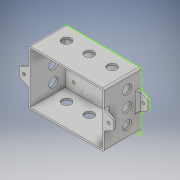
# Autodesk Inventor part: Contenedor Puente H v1.1
Saved by Autodesk Inventor 2019 (Build 230136000, 136)
## iProperties
Created: 2018-07-23
Part Number: Contenedor Puente H v1.1
Material: Genérico
Document SubType Name: Modeling
Designer: Francisco
Density: 1 g/cm^3
Appearance: Valor por defecto
Author: Francisco
Autodesk Inventor part; units mm, degrees
ref_plane "YZ Plane" through (0, 0, 0) normal (1, 0, 0) x (0, 1, 0)
ref_plane "XZ Plane" through (0, 0, 0) normal (0, 1, 0) x (-1, 0, 0)
ref_plane "XY Plane" through (0, 0, 0) normal (0, 0, 1) x (1, 0, 0)
sketch "Base" plane through (0, 0, 0) normal (0, 0, 1) x (1, 0, 0)
  line L0 (-41.5, -30) -> (41.5, -30)
  line L1 (41.5, -30) -> (41.5, -11.2361)
  line L2 (41.5, 30) -> (-41.5, 30)
  line L3 (-41.5, -30) -> (41.5, 30) construction
  line L4 (41.5, -30) -> (-41.5, 30) construction
  line L5 (-39.5, -28) -> (39.5, -28)
  line L6 (39.5, -28) -> (39.5, 28)
  line L7 (39.5, 28) -> (-39.5, 28)
  line L8 (-39.5, 28) -> (-39.5, -28)
  circle A0 centre (-30, -18.5) radius 1.35
  circle A1 centre (30, -18.5) radius 1.35
  circle A2 centre (0, 18.5) radius 1.35
  line L9 (51.5, 3.7639) -> (51.5, -3.7639)
  line L10 (41.5, 5) -> (51.5, -5) construction
  line L11 (51.5, 5) -> (41.5, -5) construction
  line L12 (42.6056, -9.4472) -> (50.3944, -5.5528)
  line L13 (50.3944, 5.5528) -> (42.6056, 9.4472)
  arc A3 (51.5, 3.7639) -> (50.3944, 5.5528) centre (49.5, 3.7639) ccw
  arc A4 (50.3944, -5.5528) -> (51.5, -3.7639) centre (49.5, -3.7639) ccw
  arc A5 (42.6056, -9.4472) -> (41.5, -11.2361) centre (43.5, -11.2361) ccw
  line L14 (41.5, 11.2361) -> (41.5, 30)
  arc A6 (41.5, 11.2361) -> (42.6056, 9.4472) centre (43.5, 11.2361) ccw
  line L15 (-41.5, -30) -> (-41.5, -11.2361)
  line L16 (-39.5, -28) -> (-39.5, 28)
  line L17 (-51.5, 3.7639) -> (-51.5, -3.7639)
  line L18 (-41.5, 5) -> (-51.5, -5) construction
  line L19 (-51.5, 5) -> (-41.5, -5) construction
  line L20 (-42.6056, -9.4472) -> (-50.3944, -5.5528)
  line L21 (-50.3944, 5.5528) -> (-42.6056, 9.4472)
  arc A7 (-50.3944, 5.5528) -> (-51.5, 3.7639) centre (-49.5, 3.7639) ccw
  arc A8 (-51.5, -3.7639) -> (-50.3944, -5.5528) centre (-49.5, -3.7639) ccw
  arc A9 (-41.5, -11.2361) -> (-42.6056, -9.4472) centre (-43.5, -11.2361) ccw
  line L22 (-41.5, 11.2361) -> (-41.5, 30)
  arc A10 (-42.6056, 9.4472) -> (-41.5, 11.2361) centre (-43.5, 11.2361) ccw
  line L23 (41.5, 11.2361) -> (41.5, -11.2361)
  line L24 (-41.5, -11.2361) -> (-41.5, 11.2361)
  circle A11 centre (-46.5, 0) radius 1.35
  circle A12 centre (46.5, 0) radius 1.35
  line L25 (-41.5, -34) -> (41.5, -34)
  line L26 (41.5, -34) -> (41.5, -11.2361)
  line L27 (41.5, 30) -> (-41.5, 30)
  line L28 (-41.5, -34) -> (41.5, 30) construction
  line L29 (41.5, -34) -> (-41.5, 30) construction
  line L30 (-39.5, -28) -> (35.5, -28)
  line L31 (35.5, -28) -> (35.5, 24)
  line L32 (35.5, 24) -> (-39.5, 24)
  line L33 (-39.5, 24) -> (-39.5, -28)
  circle A13 centre (-30, -18.5) radius 1.35
  circle A14 centre (30, -18.5) radius 1.35
  line L34 (51.5, 3.7639) -> (51.5, -3.7639)
  line L35 (41.5, 5) -> (51.5, -5) construction
  line L36 (51.5, 5) -> (41.5, -5) construction
  line L37 (42.6056, -9.4472) -> (50.3944, -5.5528)
  line L38 (50.3944, 5.5528) -> (42.6056, 9.4472)
  arc A15 (51.5, 3.7639) -> (50.3944, 5.5528) centre (49.5, 3.7639) ccw
  arc A16 (50.3944, -5.5528) -> (51.5, -3.7639) centre (49.5, -3.7639) ccw
  arc A17 (42.6056, -9.4472) -> (41.5, -11.2361) centre (43.5, -11.2361) ccw
  line L39 (41.5, 11.2361) -> (41.5, 30)
  arc A18 (41.5, 11.2361) -> (42.6056, 9.4472) centre (43.5, 11.2361) ccw
  line L40 (-51.5, -0.2361) -> (-51.5, -7.7639)
  line L41 (-41.5, 1) -> (-51.5, -9) construction
  line L42 (-51.5, 1) -> (-41.5, -9) construction
  arc A19 (-50.3944, 1.5528) -> (-51.5, -0.2361) centre (-49.5, -0.2361) ccw
  line L43 (-50.3944, 1.5528) -> (-42.6056, 5.4472)
  arc A20 (-42.6056, 5.4472) -> (-41.5, 7.2361) centre (-43.5, 7.2361) ccw
  line L44 (-41.5, 7.2361) -> (-41.5, 30)
  arc A21 (-51.5, -7.7639) -> (-50.3944, -9.5528) centre (-49.5, -7.7639) ccw
  line L45 (-42.6056, -13.4472) -> (-50.3944, -9.5528)
  arc A22 (-41.5, -15.2361) -> (-42.6056, -13.4472) centre (-43.5, -15.2361) ccw
  line L46 (-41.5, -34) -> (-41.5, -15.2361)
  line L47 (-39.5, -28) -> (-39.5, 24)
  line L48 (41.5, 11.2361) -> (41.5, -11.2361)
  line L49 (-41.5, -15.2361) -> (-41.5, 7.2361)
  circle A23 centre (-46.5, -4) radius 1.35
  circle A24 centre (46.5, 0) radius 1.35
  circle A25 centre (0, 18.5) radius 1.6
  circle A26 centre (30, -18.5) radius 1.6
  circle A27 centre (-30, -18.5) radius 1.6
  circle A28 centre (-46.5, 0) radius 1.6
  circle A29 centre (46.5, 0) radius 1.6
  point P0 (0, 0)
  point P1 (41.5, 10)
  point P2 (-41.5, 10)
  point P3 (-41.5, -10)
  point P4 (-41.5, 10)
  point P5 (0, -2)
  point P6 (41.5, 10)
  point P7 (-41.5, 10)
  point P8 (-41.5, -10)
  point P9 (-41.5, 6)
  dimension "d0" = 83
  dimension "d1" = 60
  dimension "d5" = 2.7
  dimension "d6" = 9.5
  dimension "d8" = 2.7
  dimension "d9" = 5
  dimension "d10" = 10
  dimension "d11" = 10
  dimension "d14" = 2
  dimension "d15" = 2
  dimension "d16" = 2.7
  dimension "d17" = 2.7
  dimension "d18" = 83
  dimension "d19" = 64
  dimension "d20" = 2.7
  dimension "d23" = 5
  dimension "d24" = 10
  dimension "d25" = 10
  dimension "d26" = 2
  dimension "d27" = 2
  dimension "d28" = 2.7
  dimension "d29" = 2.7
  dimension "d60" = 3.2
  dimension "d61" = 3.2
  dimension "d62" = 3.2
  dimension "d63" = 3.2
  dimension "d64" = 3.2
  constraints: 100 end point, 32 point on circle, 30 centre point, 28 point on line, 16 tangent, 14 coincident, 12 midpoint, 8 parallel, 4 equal radius, 4 perpendicular, 2 horizontal, 2 vertical, 4 other
  measures "d0" distance of L2.end L2.start
  measures "d1" distance of L2.start L0.end
  measures "d5" diameter of A0
  measures "d6" distance from line of L7 point (0, 18.5)
  measures "d8" diameter of A2
  measures "d9" distance from line of L1 point (46.5, 0)
  measures "d10" distance of L10.end L11.end
  measures "d11" distance of L11.start L10.end
  measures "d14" radius of A3
  measures "d15" radius of A6
  measures "d16" diameter of A11
  measures "d17" diameter of A12
  measures "d18" distance of L27.end L27.start
  measures "d19" distance of L27.start L25.end
  measures "d20" diameter of A13
  measures "d23" distance from line of L26 point (46.5, 0)
  measures "d24" distance of L35.end L36.end
  measures "d25" distance of L36.start L35.end
  measures "d26" radius of A15
  measures "d27" radius of A18
  measures "d28" diameter of A23
  measures "d29" diameter of A24
  measures "d60" diameter of A25
  measures "d61" diameter of A26
  measures "d62" diameter of A27
  measures "d63" diameter of A28
  measures "d64" diameter of A29
extrude "Extrusión1" add sketch "Base" along normal blind 2 contours L8 L32 L31 L5 | L31 L32 L8 L7 L6 L5 | A25 | A26 | A27
extrude "Extrusión2" add sketch "Base" along normal blind 2 contours L23 A6 L13 A3 L9 A4 L12 A5 | A9 L20 A8 L17 A19 L43 A20 L24 | A20 L43 A19 L17 A7 L21 A10 L24 | A23 | A28 | A29
extrude "Extrusión3" add sketch "Base" along normal blind 40 contours L15 L24 L22 L2 L14 L23 L1 L0
chamfer "Chaflán1" distance 2 angle 63 1 edges at (-41.5, 0, 2) measured on face at (-42, 0, 2)
mirror "Simetría1" about plane through (0, 0, 0) normal (1, 0, 0)
sketch "Boceto2" plane through (-41.5, -30, 0) normal (0, -1, 0) x (1, 0, 0)
  line L0 (2, 40) -> (81, 40) projected
  line L1 (0, 0) -> (83, 0) projected
  line L2 (41.5, 0) -> (41.5, 40)
  circle A0 centre (66.5, 14.9) radius 5
  circle A1 centre (16.5, 14.9) radius 5
  circle A2 centre (41.5, 14.9) radius 5
  dimension "d43" = 25
  dimension "d44" = 14.9
  dimension "d45" = 10
  dimension "d46" = 10
  constraints: 3 centre point, 2 end point, 1 coincident, 1 midpoint, 1 point on line, 1 symmetric about line, 1 other
  measures "d43" distance from line of L2 point (66.5, 14.9)
  measures "d44" distance from line of L1 point (66.5, 14.9)
  measures "d45" diameter of A0
  measures "d46" diameter of A2
extrude "Extrusión4" cut sketch "Boceto2" against normal blind 100
sketch "Boceto3" plane through (-41.5, -30, 40) normal (-1, 0, 0) x (0, 0, 1)
  point P0 (-40, 30)
sketch "Boceto4" plane through (-41.5, -30, 40) normal (-1, 0, 0) x (0, 0, 1)
  line L0 (-40, 30) -> (0, 30)
  line L1 (0, 0) -> (0, 60) projected
  line L2 (-40, 18.7639) -> (-40, 0) projected
  circle A0 centre (-25.1, 13) radius 5
  circle A1 centre (-25.1, 47) radius 5
  circle A2 centre (-25.1, 30) radius 5
  dimension "d49" = 14.9
  dimension "d50" = 10
  dimension "d51" = 17
  dimension "d52" = 10
  constraints: 3 centre point, 2 end point, 1 coincident, 1 midpoint, 1 point on line, 1 symmetric about line, 1 other
  measures "d49" distance from line of L2 point (-25.1, 13)
  measures "d50" diameter of A0
  measures "d51" distance from line of L0 A0.centre
  measures "d52" diameter of A2
extrude "Extrusión5" cut sketch "Boceto4" against normal blind 100
sketch "Boceto5" plane through (-41.5, -30, 40) normal (-1, 0, 0) x (0, 0, 1)
  line L0 (0, 60) -> (0, 0) projected
  line L1 (-38, 58) -> (0, 58) projected
  line L2 (-20, 58) -> (-20, 0)
  point P0 (-40, 30)
  point P1 (-20, 30)
  dimension "d55" = 20
  constraints: 2 end point, 1 point on line, 1 vertical
  measures "d55" distance from line of L0 point (-20, 30)
ref_plane "Plano de trabajo1" through (-41.5, 0, 20) normal (0, 0, 1) x (1, 0, 0)
mirror "Simetría2" about plane through (-41.5, 0, 20) normal (0, 0, 1) of "Extrusión2", "Chaflán1"
fillet "Empalme1" radius 2 4 edges at (-41.5, -30, 20) (-41.5, 30, 20) (41.5, 30, 20) (41.5, -30, 20)
chamfer "Chaflán2" distance 2 angle 63 1 edges at (41.5, 0, 38) measured on face at (42, 0, 38)
extrude "Extrusión6" cut sketch "Base" along normal blind 50 contours A12 | A25 | A26 | A27 | A28 | A29
